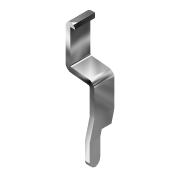
# Autodesk Inventor part: pin_1
Saved by Autodesk Inventor 2014 (Build 180170000, 170)
## iProperties
Created: 2015-10-12
Part Number: pin_1
Material: Generic
Document SubType Name: Modeling
Designer: Tom
Density: 1 g/cm^3
Appearance: Chrome - Polished
d3: 0.015 in
d4: 0.015 in
d8: 0.065 in
d9: 0.00 deg
d10: 0.005 in
d11: 0.020 in
d17: 0.020 in
d18: 0.031 in
d19: 0.100 in
d21: 0.00 deg
d22: 0.030 in
d23: 0.015 in
d24: 0.065 in
d25: 0.00 deg
d26: 0.015 in
Author: Tom
Autodesk Inventor part; units mm, degrees
note: some values were not read from the file. Chosen so that the rebuilt part matches the saved one: edges of "Fillet2".
ref_plane "YZ Plane" through (0, 0, 0) normal (1, 0, 0) x (0, 1, 0)
ref_plane "XZ Plane" through (0, 0, 0) normal (0, 1, 0) x (-1, 0, 0)
ref_plane "XY Plane" through (0, 0, 0) normal (0, 0, 1) x (1, 0, 0)
sketch "Sketch1" plane through (0, 0, 0) normal (0, 0, 1) x (1, 0, 0)
  line L0 (0.6985, 3.9665) -> (0.6985, 6.5405)
  line L1 (0.3175, 6.1595) -> (0.3175, 3.9665)
  line L2 (-1.651, 6.35) -> (-1.651, 6.731)
  line L3 (-1.27, 6.731) -> (-1.27, 9.906)
  line L4 (-1.27, 9.906) -> (-1.651, 9.906)
  line L5 (-1.651, 9.906) -> (-1.651, 6.35)
  line L6 (-0.0635, 2.0785) -> (-0.0635, 0.1905)
  line L7 (-0.0635, 0.1905) -> (0.3175, 0.1905)
  line L8 (0.3175, 0.1905) -> (0.3175, 2.0785)
  line L9 (0.6985, 3.9665) -> (0.3175, 2.0785)
  line L10 (0.3175, 3.9665) -> (-0.0635, 2.0785)
  line L11 (-1.27, 6.731) -> (0.6985, 6.5405)
  line L12 (-1.651, 6.35) -> (0.3175, 6.1595)
  point P0 (0, 0)
  dimension "d3" = 0.381
  dimension "d4" = 0.381
  constraints: 26 end point, 3 parallel
  measures "d3" distance of L2.start L2.end
  measures "d4" distance of L4.end L3.end
extrude "Extrusion1" add sketch "Sketch1" along normal blind 1.651
fillet "Fillet1" radius 0.127 2 edges at (0.3175, 6.1595, 0.8255) (-1.27, 6.731, 0.8255)
fillet "Fillet2" radius 0.508 2 edges at (-1.651, 6.35, 0.8255) (0.6985, 6.5405, 0.8255)
fillet_without_effect "Fillet3"
sketch "Sketch3" plane through (-0.0635, 0.1905, 0) normal (-1, 0, 0) x (0, 0, 1)
  line L0 (0, 0) -> (0.7874, 0)
  line L1 (0.7874, 0) -> (0.7874, 2.54)
  line L2 (0.7874, 2.54) -> (0, 2.54)
  line L3 (0, 2.54) -> (0, 0)
  point P0 (0, -0.1905)
  dimension "d18" = 0.7874
  dimension "d19" = 2.54
  constraints: 8 end point, 2 parallel, 1 horizontal, 1 perpendicular
  measures "d18" distance of L2.end L1.end
  measures "d19" distance of L1.end L0.end
extrude "Extrusion3" cut sketch "Sketch3" against normal through all
sketch "Sketch4" plane through (0, 0, 1.651) normal (0, 0, 1) x (1, 0, 0)
  line L0 (-1.651, 9.906) -> (-0.889, 9.906)
  line L1 (-0.889, 9.906) -> (-0.889, 9.525)
  line L2 (-0.889, 9.525) -> (-1.651, 9.525)
  line L3 (-1.651, 9.525) -> (-1.651, 9.906)
  point P0 (0, 0)
  dimension "d22" = 0.762
  dimension "d23" = 0.381
  constraints: 8 end point, 2 parallel, 1 horizontal, 1 perpendicular
  measures "d22" distance of L1.end L2.end
  measures "d23" distance of L0.end L1.end
extrude "Extrusion4" add sketch "Sketch4" against normal blind 1.651
fillet "Fillet4" radius 0.381 1 edges at (-1.651, 9.906, 0.8255)
fillet "Fillet5" radius 0.508 2 edges at (0.127, 0.1905, 1.651) (0.127, 0.1905, 0.7874)
body "Solid1"
